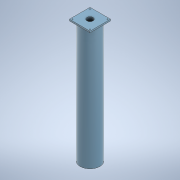
# Autodesk Inventor part: RaAxis
Saved by Autodesk Inventor 2022 (Build 260153000, 153)
## iProperties
Created: 2021-04-24
Part Number: RaAxis
Material: Generic
Document SubType Name: Modeling
Designer: Mick Veldhuis
Density: 1 g/cm^3
Appearance: Default
Author: Mick Veldhuis
Autodesk Inventor part; units mm, degrees
ref_plane "YZ Plane" through (0, 0, 0) normal (1, 0, 0) x (0, 1, 0)
ref_plane "XZ Plane" through (0, 0, 0) normal (0, 1, 0) x (-1, 0, 0)
sketch "Sketch1" plane through (0, 0, 0) normal (0, 1, 0) x (-1, 0, 0)
  circle A0 centre (0, 0) radius 65
  dimension "d0" = 130
  constraints: 1 centre point, 1 coincident
  measures "d0" diameter of A0
extrude "Beam" add sketch "Sketch1" along normal blind 800
ref_plane "Work Plane1" through (0, 800, 0) normal (0, 1, 0) x (1, 0, 0)
sketch "Sketch2" plane through (0, 800, 0) normal (0, 1, 0) x (1, 0, 0)
  line L0 (-68, 68) -> (68, 68)
  line L1 (68, 68) -> (68, -68)
  line L2 (68, -68) -> (-68, -68)
  line L3 (-68, -68) -> (-68, 68)
  line L4 (-68, 68) -> (68, -68) construction
  line L5 (68, 68) -> (-68, -68) construction
  point P0 (0, 0)
  constraints: 12 end point, 2 midpoint, 2 parallel, 1 horizontal, 1 perpendicular
extrude "Connector" add sketch "Sketch2" along normal blind 10
sketch "Sketch6" plane through (0, 810, 0) normal (0, 1, 0) x (1, 0, 0)
  circle A0 centre (0, 0) radius 20
  constraints: 1 centre point, 1 coincident
extrude "CableHole" cut sketch "Sketch6" against normal up to next
sketch "Sketch8" plane through (0, 800, 0) normal (0, -1, 0) x (1, 0, 0)
  point P0 (0, 0)
  point P1 (58, -58)
  point P2 (-58, -58)
  point P3 (-58, 58)
  point P4 (58, 58)
hole "Hole2" at (58, 800, -58) at (-58, 800, -58) at (-58, 800, 58) at (58, 800, 58) direction (0, 1, 0) diameter 6 depth 10 tip angle 118 counterbore diameter 9 counterbore depth 2
body "Solid1"
